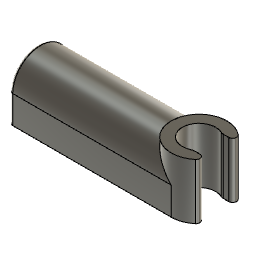
connecteur_T_boxkite v3 (Autodesk Fusion 360 design; units mm, degrees)
Autodesk Fusion 360 part; units mm, degrees
sketch "Esquisse1" plane through (0, 0, 0) normal (0, 0, 1) x (1, 0, 0)
  circle A0 centre (0, 0) radius 3
  circle A1 centre (0, 0) radius 5
  line L0 (0, 0) -> (5, 0) construction
  line L1 (1.4967, 2.6) -> (4.2708, 2.6)
  line L2 (1.4967, -2.6) -> (4.2708, -2.6)
  dimension "d1" = 6
  dimension "d2" = 10
  dimension "d3" = 2.6
  constraint coincident A0.centre A1.centre
  constraint concentric A0 A1
  constraint coincident A1 L0.end
  constraint horizontal L0
  constraint coincident A0 L1.start
  constraint coincident A1 L1.end
  constraint parallel L0 L1
  constraint symmetric L0 L1.start L2.start
  constraint symmetric L0 L1.end L2.end
  measures "d1" diameter of A0
  measures "d2" diameter of A1
  measures "d3" distance of L0 L1
extrude "Extrusion1" add sketch "Esquisse1" along normal blind 10 contours A0 A1 L1 L2 picked at (-4.3242, 0)
ref_plane "Plan de construction1" through (-4, 0, 0) normal (1, 0, 0) x (0, 1, 0)
sketch "Esquisse2" plane through (-4, 0, 0) normal (1, 0, 0) x (0, 1, 0)
  circle A0 centre (0, 5) radius 3.25
  line L0 (0, 0) -> (0, 12.3811) construction
  circle A1 centre (0, 5) radius 5
  line L1 (5, 0) -> (5, 5)
  line L2 (0, 0) -> (5, 0)
  line L3 (0, 0) -> (-5, 0)
  line L4 (-5, 0) -> (-5, 5)
  dimension "d6" = 6.5
  dimension "d7" = 5
  constraint coincident L0.start L2.start
  constraint vertical L0
  constraint coincident A0.centre L0
  constraint concentric A0 A1
  constraint coincident L0.start A1
  constraint coincident A1 L1.end
  constraint tangent A1 L1
  constraint tangent A1 L2
  constraint tangent A1 L3
  constraint perpendicular L0 L3
  constraint coincident A1 L4.end
  constraint tangent A1 L4
  measures "d6" diameter of A0
  measures "d7" distance of L0.start A0.centre
extrude "Extrusion2" add sketch "Esquisse2" against normal blind 25
extrude "Extrusion3" add 2 faces at (-4, 4.3333, 2.9167) (-4, -4.3333, 2.9167) along direction (1, 0, 0) blind 4
chamfer "Chanfrein1" distance 1 angle 45 1 edges at (-29, -3.0301, 3.8247)
fillet "Congé1" radius 0.5 1 edges at (-29, 0, 10)
fillet "Congé2" radius 0.7 2 edges at (4.2708, 2.6, 5) (4.2708, -2.6, 5)
fillet "Congé3" radius 1 2 edges at (1.4967, -2.6, 5) (1.4967, 2.6, 5)
equation "d4 = 10 mm"
equation "d7 = d4 / 2"
